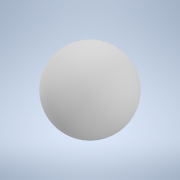
# Autodesk Inventor part: A Ball
Saved by Autodesk Inventor 2021 (Build 250183000, 183)
## iProperties
Created: 2021-03-20
Part Number: A Ball
Material: Generic
Document SubType Name: Modeling
Designer: tieub
Density: 1 g/cm^3
Appearance: Default
Author: tieub
Autodesk Inventor part; units mm, degrees
ref_plane "YZ Plane" through (0, 0, 0) normal (1, 0, 0) x (0, 1, 0)
ref_plane "XZ Plane" through (0, 0, 0) normal (0, 1, 0) x (-1, 0, 0)
ref_plane "XY Plane" through (0, 0, 0) normal (0, 0, 1) x (1, 0, 0)
sketch "Sketch3" plane through (0, 0, 0) normal (0, 0, 1) x (1, 0, 0)
  arc A0 (0, 150) -> (0, -150) centre (0, 0) ccw
  line L0 (0, 150) -> (0, -150)
  dimension "d1" = 300
  constraints: 2 end point, 2 point on circle, 1 centre point, 1 coincident, 1 vertical
  measures "d1" diameter of A0
revolve "Revolution1" add sketch "Sketch3" angle 360 about axis through (0, 150, 0) along (0, -1, 0)
body "Solid1"
